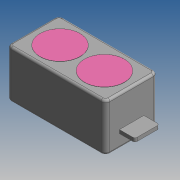
# Autodesk Inventor part: P041_Lidar
Saved by Autodesk Inventor 2021.3 (Build 253353000, 353)
## iProperties
Created: 2021-12-17
Part Number: P041_Lidar
Material: Générique
Document SubType Name: Modeling
Designer: gabri
Density: 1 g/cm^3
Appearance: Par défaut
Author: gabri
Autodesk Inventor part; units mm, degrees
ref_plane "YZ Plane" through (0, 0, 0) normal (1, 0, 0) x (0, 1, 0)
ref_plane "XZ Plane" through (0, 0, 0) normal (0, 1, 0) x (-1, 0, 0)
ref_plane "XY Plane" through (0, 0, 0) normal (0, 0, 1) x (1, 0, 0)
sketch "Sketch2" plane through (0, 0, 0) normal (0, 0, 1) x (1, 0, 0)
  line L0 (22.25, -11.75) -> (-22.25, -11.75)
  line L1 (-22.25, -11.75) -> (-22.25, 11.75)
  line L2 (-22.25, 11.75) -> (22.25, 11.75)
  line L3 (22.25, 11.75) -> (22.25, -11.75)
  line L4 (22.25, -11.75) -> (-22.25, 11.75) construction
  line L5 (-22.25, -11.75) -> (22.25, 11.75) construction
  point P0 (0, 0)
  dimension "d0" = 44.5
  dimension "d1" = 23.5
  constraints: 12 end point, 2 midpoint, 2 parallel, 1 horizontal, 1 perpendicular
  measures "d0" distance between parallel lines of L3 L1
  measures "d1" distance between parallel lines of L0 L2
extrude "Extrusion1" add sketch "Sketch2" along normal blind 21.5
sketch "Sketch3" plane through (22.25, -11.75, 0) normal (1, 0, 0) x (0, 0, -1)
  line L0 (-7.5, 17.25) -> (-5.9, 17.25)
  line L1 (-5.9, 17.25) -> (-5.9, 6.25)
  line L2 (-5.9, 6.25) -> (-7.5, 6.25)
  line L3 (-7.5, 6.25) -> (-7.5, 17.25)
  line L4 (-21.5, 0) -> (-21.5, 23.5) construction
  line L5 (0, 23.5) -> (-21.5, 23.5) construction
  point P0 (0, 11.75)
  dimension "d4" = 11
  dimension "d5" = 1.6
  dimension "d6" = 14
  dimension "d7" = 6.25
  dimension "d8" = 23.5
  constraints: 8 end point, 2 parallel, 1 horizontal, 1 perpendicular
  measures "d4" distance between parallel lines of L2 L0
  measures "d5" distance between parallel lines of L1 L3
  measures "d6" distance between parallel lines of L4 L3
  measures "d7" distance between parallel lines of L5 L0
  measures "d8" distance of L4.start L4.end
extrude "Extrusion2" add sketch "Sketch3" along normal blind 7
sketch "Sketch4" plane through (0, 0, 21.5) normal (0, 0, 1) x (1, 0, 0)
  line L0 (22.25, 11.75) -> (-22.25, 11.75) construction
  line L1 (-22.25, 11.75) -> (-22.25, -11.75) construction
  line L2 (-22.25, -11.75) -> (22.25, -11.75) construction
  line L3 (22.25, -11.75) -> (22.25, 11.75) construction
  circle A0 centre (-10, 0) radius 9
  circle A1 centre (10, 0) radius 9
  line L4 (0, 16.45) -> (0, -16.45) construction
  line L5 (-33.55, 0) -> (45.55, 0) construction
  point P0 (0, 0)
  dimension "d11" = 18
  dimension "d12" = 10
  dimension "d13" = 18
  dimension "d14" = 10
  constraints: 2 centre point, 2 point on line
  measures "d11" diameter of A0
  measures "d12" distance from line of L4 A0.centre
  measures "d13" diameter of A1
  measures "d14" distance from line of L4 A1.centre
extrude "Extrusion3" add sketch "Sketch4" along normal blind 0.1
fillet "Fillet1" radius 2 4 edges at (-22.25, 11.75, 10.75) (22.25, 11.75, 10.75) (22.25, -11.75, 10.75) (-22.25, -11.75, 10.75)
fillet "Fillet2" radius 1 18 edges at (-21.6642, 11.1642, 21.5) (-22.25, 0, 21.5) (-21.6642, -11.1642, 21.5) (0, -11.75, 21.5) (21.6642, -11.1642, 21.5) (22.25, 0, 21.5) (21.6642, 11.1642, 21.5) (0, 11.75, 21.5) (-21.6642, 11.1642, 0) (-22.25, 0, 0) (-21.6642, -11.1642, 0) (0, -11.75, 0) (21.6642, -11.1642, 0) (22.25, 0, 0) (21.6642, 11.1642, 0) (0, 11.75, 0) (29.25, 5.5, 6.7) (29.25, -5.5, 6.7)
sketch "Sketch5" plane through (-20.25, 11.75, 1) normal (0, 1, 0) x (1, 0, 0)
  point P0 (20.25, 1)
equation "\"d7\" = -0.5 * d4 + 0.5 * d8"
body "Solid1"
